output_shaft_test_new_screw v2 (Autodesk Fusion 360 design; units mm, degrees)
Autodesk Fusion 360 part; units mm, degrees
sketch "Sketch1" plane through (0, 0, 0) normal (0, 0, 1) x (1, 0, 0)
  circle A0 centre (0, 0) radius 27.5
  circle A1 centre (0, 0) radius 34
  circle A2 centre (0, 0) radius 27.5 construction
  line L0 (0, 0) -> (0, 34) construction
  circle A3 centre (0, 27.5) radius 3.65
  circle A4 centre (0, 0) radius 21.75 construction
  circle A5 centre (-10.875, 18.8361) radius 3.5
  circle A6 centre (0, 0) radius 16.5
  line L1 (0, 0) -> (-10.875, 18.8361) construction
  line L2 (0, 0) -> (-23.8157, 13.75) construction
  circle A7 centre (-21.75, 0) radius 3.5
  circle A8 centre (-10.875, -18.8361) radius 3.5
  circle A9 centre (10.875, -18.8361) radius 3.5
  circle A10 centre (21.75, 0) radius 3.5
  circle A11 centre (10.875, 18.8361) radius 3.5
  circle A12 centre (0, 27.5) radius 2.25
  circle A13 centre (-23.8157, 13.75) radius 2.25
  circle A14 centre (-23.8157, -13.75) radius 2.25
  circle A15 centre (0, -27.5) radius 2.25
  circle A16 centre (23.8157, -13.75) radius 2.25
  circle A17 centre (23.8157, 13.75) radius 2.25
  circle A18 centre (-23.8157, 13.75) radius 3.65
  circle A19 centre (-23.8157, -13.75) radius 3.65
  circle A20 centre (0, -27.5) radius 3.65
  circle A21 centre (23.8157, -13.75) radius 3.65
  circle A22 centre (23.8157, 13.75) radius 3.65
  dimension "d1" = 55
  dimension "d3" = 55
  dimension "d4" = 7.3
  dimension "d7" = 7
  dimension "d8" = 33
  dimension "d9" = 43.5
  dimension "d10" = 60
  dimension "d11" = 30
  dimension "d13" = 360
  dimension "d15" = 68
  dimension "d21" = 4.5
  dimension "d23" = 360
  dimension "d30" = 360
  constraint coincident A0.centre A1.centre
  constraint concentric A0 A2
  constraint coincident A1 L0.end
  constraint vertical L0
  constraint coincident L0 A3.centre
  constraint coincident A2 A3.centre
  constraint coincident A4 A5.centre
  constraint coincident A5.centre L1.end
  constraint concentric A3 A12
  measures "d1" diameter of A0
  measures "d3" diameter of A2
  measures "d4" diameter of A3
  measures "d7" diameter of A5
  measures "d8" diameter of A6
  measures "d9" diameter of A4
  measures "d10" angle of L0 L2
  measures "d11" angle of L0 L1
  measures "d15" diameter of A1
  measures "d21" diameter of A12
extrude "Extrude1" add sketch "Sketch1" against normal blind 7 contours A0 A3 A18 A19 A20 A21 A22 | A0 A17 A22 | A0 A17 A22 | A0 A16 A21 | A0 A16 A21 | A0 A3 A12 | A0 A3 A12 | A0 A15 A20 | A0 A15 A20 | A0 A13 A18 | A0 A13 A18 | A0 A14 A19 | A0 A14 A19 | A1 | A5 | A7 | A8 | A9 | A10 | A11
extrude "Extrude2" add sketch "Sketch1" along normal blind 10 contours A0 A3 A18 A19 A20 A21 A22
extrude "Extrude3" cut sketch "Sketch1" against normal blind 5 contours A0 A17 A22 | A0 A17 A22 | A0 A16 A21 | A0 A16 A21 | A0 A17 | A0 A17 | A0 A16 | A0 A16 | A0 A3 A12 | A0 A3 A12 | A0 A15 A20 | A0 A15 A20 | A0 A12 | A0 A15 | A0 A15 | A0 A13 A18 | A0 A13 A18 | A0 A14 A19 | A0 A14 A19 | A0 A13 | A0 A13 | A0 A14 | A0 A14 picked at (0.0546, 26.7452)
sketch "Sketch2" plane through (0, 0, -7) normal (0, 0, -1) x (1, 0, 0)
  circle A0 centre (0, -27.5) radius 2.25
  circle A1 centre (-23.8157, -13.75) radius 2.25
  circle A2 centre (23.8157, -13.75) radius 2.25
  circle A3 centre (0, 27.5) radius 2.25
  circle A4 centre (23.8157, 13.75) radius 2.25
  circle A5 centre (0, 0) radius 16.5
  circle A6 centre (-23.8157, 13.75) radius 2.25
  circle A7 centre (0, 0) radius 34
  circle A8 centre (0, 0) radius 18.8
  dimension "d26" = 37.6
  constraint concentric A5 A8
  measures "d26" diameter of A8
extrude "Extrude4" cut sketch "Sketch2" against normal blind 7 contours A8
sketch "Sketch3" plane through (0, 0, 10) normal (0, 0, 1) x (-1, 0, 0)
  circle A0 centre (-10.875, -18.8361) radius 3.5
  circle A1 centre (-21.75, 0) radius 3.5
  circle A2 centre (0, 0) radius 16.5
  circle A3 centre (10.875, 18.8361) radius 3.5
  circle A4 centre (-10.875, 18.8361) radius 3.5
  circle A5 centre (21.75, 0) radius 3.5
  circle A6 centre (10.875, -18.8361) radius 3.5
  arc A7 (-3.642, 27.2578) -> (-21.7849, 16.7829) centre (0, 0) ccw
  arc A8 (-25.4269, 10.4749) -> (-21.7849, 16.7829) centre (-23.8157, 13.75) ccw
  arc A9 (-25.4269, 10.4749) -> (-25.4269, -10.4749) centre (0, 0) ccw
  arc A10 (-21.7849, -16.7829) -> (-25.4269, -10.4749) centre (-23.8157, -13.75) ccw
  arc A11 (-21.7849, -16.7829) -> (-3.642, -27.2578) centre (0, 0) ccw
  arc A12 (3.642, -27.2578) -> (-3.642, -27.2578) centre (0, -27.5) ccw
  arc A13 (3.642, -27.2578) -> (21.7849, -16.7829) centre (0, 0) ccw
  arc A14 (25.4269, -10.4749) -> (21.7849, -16.7829) centre (23.8157, -13.75) ccw
  arc A15 (25.4269, -10.4749) -> (25.4269, 10.4749) centre (0, 0) ccw
  arc A16 (21.7849, 16.7829) -> (25.4269, 10.4749) centre (23.8157, 13.75) ccw
  arc A17 (21.7849, 16.7829) -> (3.642, 27.2578) centre (0, 0) ccw
  arc A18 (-3.642, 27.2578) -> (3.642, 27.2578) centre (0, 27.5) ccw
extrude "Extrude5" add sketch "Sketch3" against normal blind 10 contours A0 | A1 | A3 | A4 | A5 | A6
extrude "Extrude6" cut sketch "Sketch3" against normal blind 9 contours A0 | A1 | A3 | A4 | A5 | A6
sketch "Sketch4" plane through (0, 0, 10) normal (0, 0, 1) x (-1, 0, 0)
  circle A0 centre (-10.875, 18.8361) radius 3.5
  circle A1 centre (10.875, -18.8361) radius 3.5
  circle A2 centre (10.875, 18.8361) radius 3.5
  circle A3 centre (-21.75, 0) radius 3.5
  circle A4 centre (-10.875, -18.8361) radius 3.5
  circle A5 centre (21.75, 0) radius 3.5
  circle A6 centre (0, 0) radius 16.5
  arc A7 (-3.642, 27.2578) -> (-21.7849, 16.7829) centre (0, 0) ccw
  arc A8 (-25.4269, 10.4749) -> (-21.7849, 16.7829) centre (-23.8157, 13.75) ccw
  arc A9 (-25.4269, 10.4749) -> (-25.4269, -10.4749) centre (0, 0) ccw
  arc A10 (-21.7849, -16.7829) -> (-25.4269, -10.4749) centre (-23.8157, -13.75) ccw
  arc A11 (-21.7849, -16.7829) -> (-3.642, -27.2578) centre (0, 0) ccw
  arc A12 (3.642, -27.2578) -> (-3.642, -27.2578) centre (0, -27.5) ccw
  arc A13 (3.642, -27.2578) -> (21.7849, -16.7829) centre (0, 0) ccw
  arc A14 (25.4269, -10.4749) -> (21.7849, -16.7829) centre (23.8157, -13.75) ccw
  arc A15 (25.4269, -10.4749) -> (25.4269, 10.4749) centre (0, 0) ccw
  arc A16 (21.7849, 16.7829) -> (25.4269, 10.4749) centre (23.8157, 13.75) ccw
  arc A17 (21.7849, 16.7829) -> (3.642, 27.2578) centre (0, 0) ccw
  arc A18 (-3.642, 27.2578) -> (3.642, 27.2578) centre (0, 27.5) ccw
  circle A19 centre (10.875, -18.8361) radius 2.5
  circle A20 centre (21.75, 0) radius 2.5
  circle A21 centre (10.875, 18.8361) radius 2.5
  circle A22 centre (-10.875, 18.8361) radius 2.5
  circle A23 centre (-21.75, 0) radius 2.5
  circle A24 centre (-10.875, -18.8361) radius 2.5
  dimension "d35" = 5
  dimension "d37" = 360
  constraint concentric A1 A19
  measures "d35" diameter of A19
extrude "Extrude7" add sketch "Sketch4" against normal blind 10 contours A0 | A1 | A2 | A3 | A4 | A5
extrude "Extrude8" cut sketch "Sketch4" against normal blind 17 contours A19 | A20 | A21 | A22 | A23 | A24
equation "d3 = ( 27.5 * 2 ) * 1 mm"
equation "d9 = 33 mm + 10.5 mm"
equation "d11 = d10 / 2"
